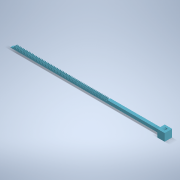
# Autodesk Inventor part: 도면
Saved by Autodesk Inventor 2021 (Build 250183000, 183)
## iProperties
Created: 2021-08-27
Part Number: 도면
Material: 티타늄
Document SubType Name: Modeling
Designer: Dongyoon
Density: 4.51 g/cm^3
Appearance: 티타늄
Author: Dongyoon
Autodesk Inventor part; units mm, degrees
ref_plane "YZ Plane" through (0, 0, 0) normal (1, 0, 0) x (0, 1, 0)
ref_plane "XZ Plane" through (0, 0, 0) normal (0, 1, 0) x (-1, 0, 0)
ref_plane "XY Plane" through (0, 0, 0) normal (0, 0, 1) x (1, 0, 0)
sketch "스케치3" plane through (0, 0, 0) normal (0, 0, 1) x (1, 0, 0)
  line L0 (0, 0) -> (0, -2)
  line L1 (0, -2) -> (-200, -2)
  line L2 (-200, -2) -> (-200, 2)
  line L3 (-200, 2) -> (0, 2)
  line L4 (0, 2) -> (0, 0)
  line L5 (-70, 2) -> (-70, -2)
  line L6 (-70, 2) -> (-71.5, 0)
  line L7 (-71.5, 0) -> (-72, 0)
  line L8 (-72, 0) -> (-72, 2)
  line L9 (-72, 2) -> (-72.5, 2)
  line L10 (-72.5, 2) -> (-73.5, 0)
  line L11 (-73.5, 0) -> (-74, 0)
  line L12 (-74, 0) -> (-74, 2)
  line L13 (-200, -2) -> (-196, 0)
  line L14 (-76, 0) -> (-76, 2)
  line L15 (-75.5, 0) -> (-76, 0)
  line L16 (-74.5, 2) -> (-75.5, 0)
  line L17 (-74, 2) -> (-74.5, 2)
  line L18 (-78, 0) -> (-78, 2)
  line L19 (-77.5, 0) -> (-78, 0)
  line L20 (-76.5, 2) -> (-77.5, 0)
  line L21 (-76, 2) -> (-76.5, 2)
  line L22 (-80, 0) -> (-80, 2)
  line L23 (-79.5, 0) -> (-80, 0)
  line L24 (-78.5, 2) -> (-79.5, 0)
  line L25 (-78, 2) -> (-78.5, 2)
  line L26 (-82, 0) -> (-82, 2)
  line L27 (-81.5, 0) -> (-82, 0)
  line L28 (-80.5, 2) -> (-81.5, 0)
  line L29 (-80, 2) -> (-80.5, 2)
  line L30 (-84, 0) -> (-84, 2)
  line L31 (-83.5, 0) -> (-84, 0)
  line L32 (-82.5, 2) -> (-83.5, 0)
  line L33 (-82, 2) -> (-82.5, 2)
  line L34 (-86, 0) -> (-86, 2)
  line L35 (-85.5, 0) -> (-86, 0)
  line L36 (-84.5, 2) -> (-85.5, 0)
  line L37 (-84, 2) -> (-84.5, 2)
  line L38 (-88, 0) -> (-88, 2)
  line L39 (-87.5, 0) -> (-88, 0)
  line L40 (-86.5, 2) -> (-87.5, 0)
  line L41 (-86, 2) -> (-86.5, 2)
  line L42 (-90, 0) -> (-90, 2)
  line L43 (-89.5, 0) -> (-90, 0)
  line L44 (-88.5, 2) -> (-89.5, 0)
  line L45 (-88, 2) -> (-88.5, 2)
  line L46 (-92, 0) -> (-92, 2)
  line L47 (-91.5, 0) -> (-92, 0)
  line L48 (-90.5, 2) -> (-91.5, 0)
  line L49 (-90, 2) -> (-90.5, 2)
  line L50 (-94, 0) -> (-94, 2)
  line L51 (-93.5, 0) -> (-94, 0)
  line L52 (-92.5, 2) -> (-93.5, 0)
  line L53 (-92, 2) -> (-92.5, 2)
  line L54 (-96, 0) -> (-96, 2)
  line L55 (-95.5, 0) -> (-96, 0)
  line L56 (-94.5, 2) -> (-95.5, 0)
  line L57 (-94, 2) -> (-94.5, 2)
  line L58 (-98, 0) -> (-98, 2)
  line L59 (-97.5, 0) -> (-98, 0)
  line L60 (-96.5, 2) -> (-97.5, 0)
  line L61 (-96, 2) -> (-96.5, 2)
  line L62 (-100, 0) -> (-100, 2)
  line L63 (-99.5, 0) -> (-100, 0)
  line L64 (-98.5, 2) -> (-99.5, 0)
  line L65 (-98, 2) -> (-98.5, 2)
  line L66 (-102, 0) -> (-102, 2)
  line L67 (-101.5, 0) -> (-102, 0)
  line L68 (-100.5, 2) -> (-101.5, 0)
  line L69 (-100, 2) -> (-100.5, 2)
  line L70 (-104, 0) -> (-104, 2)
  line L71 (-103.5, 0) -> (-104, 0)
  line L72 (-102.5, 2) -> (-103.5, 0)
  line L73 (-102, 2) -> (-102.5, 2)
  line L74 (-106, 0) -> (-106, 2)
  line L75 (-105.5, 0) -> (-106, 0)
  line L76 (-104.5, 2) -> (-105.5, 0)
  line L77 (-104, 2) -> (-104.5, 2)
  line L78 (-108, 0) -> (-108, 2)
  line L79 (-107.5, 0) -> (-108, 0)
  line L80 (-106.5, 2) -> (-107.5, 0)
  line L81 (-106, 2) -> (-106.5, 2)
  line L82 (-110, 0) -> (-110, 2)
  line L83 (-109.5, 0) -> (-110, 0)
  line L84 (-108.5, 2) -> (-109.5, 0)
  line L85 (-108, 2) -> (-108.5, 2)
  line L86 (-112, 0) -> (-112, 2)
  line L87 (-111.5, 0) -> (-112, 0)
  line L88 (-110.5, 2) -> (-111.5, 0)
  line L89 (-110, 2) -> (-110.5, 2)
  line L90 (-114, 0) -> (-114, 2)
  line L91 (-113.5, 0) -> (-114, 0)
  line L92 (-112.5, 2) -> (-113.5, 0)
  line L93 (-112, 2) -> (-112.5, 2)
  line L94 (-116, 0) -> (-116, 2)
  line L95 (-115.5, 0) -> (-116, 0)
  line L96 (-114.5, 2) -> (-115.5, 0)
  line L97 (-114, 2) -> (-114.5, 2)
  line L98 (-118, 0) -> (-118, 2)
  line L99 (-117.5, 0) -> (-118, 0)
  line L100 (-116.5, 2) -> (-117.5, 0)
  line L101 (-116, 2) -> (-116.5, 2)
  line L102 (-120, 0) -> (-120, 2)
  line L103 (-119.5, 0) -> (-120, 0)
  line L104 (-118.5, 2) -> (-119.5, 0)
  line L105 (-118, 2) -> (-118.5, 2)
  line L106 (-122, 0) -> (-122, 2)
  line L107 (-121.5, 0) -> (-122, 0)
  line L108 (-120.5, 2) -> (-121.5, 0)
  line L109 (-120, 2) -> (-120.5, 2)
  line L110 (-124, 0) -> (-124, 2)
  line L111 (-123.5, 0) -> (-124, 0)
  line L112 (-122.5, 2) -> (-123.5, 0)
  line L113 (-122, 2) -> (-122.5, 2)
  line L114 (-126, 0) -> (-126, 2)
  line L115 (-125.5, 0) -> (-126, 0)
  line L116 (-124.5, 2) -> (-125.5, 0)
  line L117 (-124, 2) -> (-124.5, 2)
  line L118 (-128, 0) -> (-128, 2)
  line L119 (-127.5, 0) -> (-128, 0)
  line L120 (-126.5, 2) -> (-127.5, 0)
  line L121 (-126, 2) -> (-126.5, 2)
  line L122 (-130, 0) -> (-130, 2)
  line L123 (-129.5, 0) -> (-130, 0)
  line L124 (-128.5, 2) -> (-129.5, 0)
  line L125 (-128, 2) -> (-128.5, 2)
  line L126 (-132, 0) -> (-132, 2)
  line L127 (-131.5, 0) -> (-132, 0)
  line L128 (-130.5, 2) -> (-131.5, 0)
  line L129 (-130, 2) -> (-130.5, 2)
  line L130 (-134, 0) -> (-134, 2)
  line L131 (-133.5, 0) -> (-134, 0)
  line L132 (-132.5, 2) -> (-133.5, 0)
  line L133 (-132, 2) -> (-132.5, 2)
  line L134 (-136, 0) -> (-136, 2)
  line L135 (-135.5, 0) -> (-136, 0)
  line L136 (-134.5, 2) -> (-135.5, 0)
  line L137 (-134, 2) -> (-134.5, 2)
  line L138 (-138, 0) -> (-138, 2)
  line L139 (-137.5, 0) -> (-138, 0)
  line L140 (-136.5, 2) -> (-137.5, 0)
  line L141 (-136, 2) -> (-136.5, 2)
  line L142 (-140, 0) -> (-140, 2)
  line L143 (-139.5, 0) -> (-140, 0)
  line L144 (-138.5, 2) -> (-139.5, 0)
  line L145 (-138, 2) -> (-138.5, 2)
  line L146 (-142, 0) -> (-142, 2)
  line L147 (-141.5, 0) -> (-142, 0)
  line L148 (-140.5, 2) -> (-141.5, 0)
  line L149 (-140, 2) -> (-140.5, 2)
  line L150 (-144, 0) -> (-144, 2)
  line L151 (-143.5, 0) -> (-144, 0)
  line L152 (-142.5, 2) -> (-143.5, 0)
  line L153 (-142, 2) -> (-142.5, 2)
  line L154 (-146, 0) -> (-146, 2)
  line L155 (-145.5, 0) -> (-146, 0)
  line L156 (-144.5, 2) -> (-145.5, 0)
  line L157 (-144, 2) -> (-144.5, 2)
  line L158 (-148, 0) -> (-148, 2)
  line L159 (-147.5, 0) -> (-148, 0)
  line L160 (-146.5, 2) -> (-147.5, 0)
  line L161 (-146, 2) -> (-146.5, 2)
  line L162 (-150, 0) -> (-150, 2)
  line L163 (-149.5, 0) -> (-150, 0)
  line L164 (-148.5, 2) -> (-149.5, 0)
  line L165 (-148, 2) -> (-148.5, 2)
  line L166 (-152, 0) -> (-152, 2)
  line L167 (-151.5, 0) -> (-152, 0)
  line L168 (-150.5, 2) -> (-151.5, 0)
  line L169 (-150, 2) -> (-150.5, 2)
  line L170 (-154, 0) -> (-154, 2)
  line L171 (-153.5, 0) -> (-154, 0)
  line L172 (-152.5, 2) -> (-153.5, 0)
  line L173 (-152, 2) -> (-152.5, 2)
  line L174 (-156, 0) -> (-156, 2)
  line L175 (-155.5, 0) -> (-156, 0)
  line L176 (-154.5, 2) -> (-155.5, 0)
  line L177 (-154, 2) -> (-154.5, 2)
  line L178 (-158, 0) -> (-158, 2)
  line L179 (-157.5, 0) -> (-158, 0)
  line L180 (-156.5, 2) -> (-157.5, 0)
  line L181 (-156, 2) -> (-156.5, 2)
  line L182 (-160, 0) -> (-160, 2)
  line L183 (-159.5, 0) -> (-160, 0)
  line L184 (-158.5, 2) -> (-159.5, 0)
  line L185 (-158, 2) -> (-158.5, 2)
  line L186 (-162, 0) -> (-162, 2)
  line L187 (-161.5, 0) -> (-162, 0)
  line L188 (-160.5, 2) -> (-161.5, 0)
  line L189 (-160, 2) -> (-160.5, 2)
  line L190 (-164, 0) -> (-164, 2)
  line L191 (-163.5, 0) -> (-164, 0)
  line L192 (-162.5, 2) -> (-163.5, 0)
  line L193 (-162, 2) -> (-162.5, 2)
  line L194 (-166, 0) -> (-166, 2)
  line L195 (-165.5, 0) -> (-166, 0)
  line L196 (-164.5, 2) -> (-165.5, 0)
  line L197 (-164, 2) -> (-164.5, 2)
  line L198 (-168, 0) -> (-168, 2)
  line L199 (-167.5, 0) -> (-168, 0)
  line L200 (-166.5, 2) -> (-167.5, 0)
  line L201 (-166, 2) -> (-166.5, 2)
  line L202 (-170, 0) -> (-170, 2)
  line L203 (-169.5, 0) -> (-170, 0)
  line L204 (-168.5, 2) -> (-169.5, 0)
  line L205 (-168, 2) -> (-168.5, 2)
  line L206 (-172, 0) -> (-172, 2)
  line L207 (-171.5, 0) -> (-172, 0)
  line L208 (-170.5, 2) -> (-171.5, 0)
  line L209 (-170, 2) -> (-170.5, 2)
  line L210 (-174, 0) -> (-174, 2)
  line L211 (-173.5, 0) -> (-174, 0)
  line L212 (-172.5, 2) -> (-173.5, 0)
  line L213 (-172, 2) -> (-172.5, 2)
  line L214 (-176, 0) -> (-176, 2)
  line L215 (-175.5, 0) -> (-176, 0)
  line L216 (-174.5, 2) -> (-175.5, 0)
  line L217 (-174, 2) -> (-174.5, 2)
  line L218 (-178, 0) -> (-178, 2)
  line L219 (-177.5, 0) -> (-178, 0)
  line L220 (-176.5, 2) -> (-177.5, 0)
  line L221 (-176, 2) -> (-176.5, 2)
  line L222 (-180, 0) -> (-180, 2)
  line L223 (-179.5, 0) -> (-180, 0)
  line L224 (-178.5, 2) -> (-179.5, 0)
  line L225 (-178, 2) -> (-178.5, 2)
  line L226 (-182, 0) -> (-182, 2)
  line L227 (-181.5, 0) -> (-182, 0)
  line L228 (-180.5, 2) -> (-181.5, 0)
  line L229 (-180, 2) -> (-180.5, 2)
  line L230 (-184, 0) -> (-184, 2)
  line L231 (-183.5, 0) -> (-184, 0)
  line L232 (-182.5, 2) -> (-183.5, 0)
  line L233 (-182, 2) -> (-182.5, 2)
  line L234 (-186, 0) -> (-186, 2)
  line L235 (-185.5, 0) -> (-186, 0)
  line L236 (-184.5, 2) -> (-185.5, 0)
  line L237 (-184, 2) -> (-184.5, 2)
  line L238 (-188, 0) -> (-188, 2)
  line L239 (-187.5, 0) -> (-188, 0)
  line L240 (-186.5, 2) -> (-187.5, 0)
  line L241 (-186, 2) -> (-186.5, 2)
  line L242 (-190, 0) -> (-190, 2)
  line L243 (-189.5, 0) -> (-190, 0)
  line L244 (-188.5, 2) -> (-189.5, 0)
  line L245 (-188, 2) -> (-188.5, 2)
  line L246 (-192, 0) -> (-192, 2)
  line L247 (-191.5, 0) -> (-192, 0)
  line L248 (-190.5, 2) -> (-191.5, 0)
  line L249 (-190, 2) -> (-190.5, 2)
  line L250 (-194, 0) -> (-194, 2)
  line L251 (-193.5, 0) -> (-194, 0)
  line L252 (-192.5, 2) -> (-193.5, 0)
  line L253 (-192, 2) -> (-192.5, 2)
  line L254 (-196, 0) -> (-196, 2)
  line L255 (-195.5, 0) -> (-196, 0)
  line L256 (-194.5, 2) -> (-195.5, 0)
  line L257 (-194, 2) -> (-194.5, 2)
  dimension "d1018" = 200
  dimension "d1019" = 4
  dimension "d1020" = 2
  dimension "d1040" = 70
  dimension "d1041" = 0.5
  dimension "d1042" = 0.5
  dimension "d1043" = 0.5
  dimension "d1044" = 2
  dimension "d1045" = 2
  dimension "d1046" = 4
  dimension "d1047" = 2
  dimension "d1050" = 2
  constraints: 514 end point, 305 horizontal alignment, 123 collinear, 122 parallel, 5 perpendicular, 4 point on line, 2 vertical, 1 horizontal, 6 other
  measures "d1018" distance of L0.end L1.end
  measures "d1019" distance of L1.end L2.end
  measures "d1020" distance of L0.start L0.end
  measures "d1040" distance between parallel lines of L4 L5
  measures "d1041" distance of L9.end L8.end
  measures "d1042" distance of L6.end L7.end
  measures "d1043" distance of L10.end L11.end
  measures "d1044" horizontal distance of L5.start L7.end
  measures "d1045" distance of L8.end L12.end
  measures "d1046" horizontal distance of L1.end L13.end
  measures "d1047" distance from line of L1 L13.end
  measures "d1050" distance of L11.end L14.start
extrude "돌출3" add sketch "스케치3" along normal mid plane 4 contours L0 L1 L5 L3 L4 | L1 L13 L255 L256 L3 L250 L251 L252 L246 L247 L248 L242 L243 L244 L238 L239 L240 L234 L235 L236 L230 L231 L232 L226 L227 L228 L222 L223 L224 L218 L219 L220 L214 L215 L216 L210 L211 L212 L206 L207 L208 L202 L203 L204 L198 L199 L200 L194 L195 L196 L190 L191 L192 L186 L187 L188 L182 L183 L184 L178 L179 L180 L174 L175 L176 L170 L171 L172 L166 L167 L168 L162 L163 L164 L158 L159 L160 L154 L155 L156 L150 L151 L152 L146 L147 L148 L142 L143 L144 L138 L139 L140 L134 L135 L136 L130 L131 L132 L126 L127 L128 L122 L123 L124 L118 L119 L120 L114 L115 L116 L110 L111 L112 L106 L107 L108 L102 L103 L104 L98 L99 L100 L94 L95 L96 L90 L91 L92 L86 L87 L88 L82 L83 L84 L78 L79 L80 L74 L75 L76 L70 L71 L72 L66 L67 L68 L62 L63 L64 L58 L59 L60 L54 L55 L56 L50 L51 L52 L46 L47 L48 L42 L43 L44 L38 L39 L40 L34 L35 L36 L30 L31 L32 L26 L27 L28 L22 L23 L24 L18 L19 L20 L14 L15 L16 L12 L11 L10 L8 L7 L6 L5
sketch "스케치4" plane through (0, 0, 0) normal (0, 0, 1) x (1, 0, 0)
  line L0 (0, 0) -> (0, 5)
  line L1 (0, 5) -> (10, 5)
  line L2 (10, 5) -> (10, -5)
  line L3 (10, -5) -> (0, -5)
  line L4 (0, -5) -> (0, 0)
  line L5 (0, -2) -> (0, 2) projected
  dimension "d1023" = 10
  dimension "d1024" = 10
  dimension "d1025" = 5
  constraints: 10 end point, 3 perpendicular, 1 collinear, 1 point on line, 1 vertical
  measures "d1023" distance of L1.end L2.end
  measures "d1024" distance of L2.end L3.end
  measures "d1025" distance of L3.end L0.start
extrude "돌출4" add sketch "스케치4" along normal mid plane 10
sketch "스케치6" plane through (0, 0, 0) normal (0, 0, 1) x (1, 0, 0)
  line L0 (0, 5) -> (10, 5) projected
  line L1 (10, -5) -> (0, -5) projected
  line L2 (3, 5) -> (7, 5)
  line L3 (7, 5) -> (7, -5)
  line L4 (7, -5) -> (3, -5)
  line L5 (3, -5) -> (3, 5)
  line L6 (0, -5) -> (0, 5) projected
  line L7 (3, 5) -> (5, 4)
  line L8 (5, 4) -> (5, 3.5)
  line L9 (5, 3.5) -> (3, 3.5)
  line L10 (3, 3.5) -> (3, 3)
  line L11 (3, 3) -> (5, 2)
  line L12 (5, 2) -> (5, 1.5)
  line L13 (5, 1.5) -> (3, 1.5)
  line L14 (3, 1.5) -> (3, 1)
  line L15 (3, 1) -> (5, 0)
  line L16 (5, 0) -> (5, -0.5)
  line L17 (5, -0.5) -> (3, -0.5)
  line L18 (3, -0.5) -> (3, -1)
  line L19 (3, -1) -> (5, -2)
  line L20 (5, -2) -> (5, -2.5)
  line L21 (5, -2.5) -> (3, -2.5)
  line L22 (3, -2.5) -> (3, -3)
  line L23 (3, -3) -> (5, -4)
  line L24 (5, -4) -> (5, -4.5)
  line L25 (5, -4.5) -> (3, -4.5)
  point P0 (0, 0)
  dimension "d1055" = 3
  dimension "d1056" = 4
  dimension "d1057" = 0.5
  dimension "d1058" = 0.5
  dimension "d1059" = 0.5
  dimension "d1060" = 2
  dimension "d1061" = 2
  dimension "d1062" = 2
  dimension "d1063" = 0.5
  dimension "d1064" = 0.5
  dimension "d1065" = 0.5
  dimension "d1066" = 0.5
  dimension "d1067" = 0.5
  dimension "d1068" = 0.5
  constraints: 46 end point, 7 point on line, 3 perpendicular, 2 parallel, 1 horizontal, 1 vertical
  measures "d1055" distance between parallel lines of L6 L5
  measures "d1056" distance between parallel lines of L5 L3
  measures "d1057" distance of L7.end L8.end
  measures "d1058" distance of L9.end L10.end
  measures "d1059" distance of L11.end L12.end
  measures "d1060" distance of L10.end L2.start
  measures "d1061" distance of L11.end L7.end
  measures "d1062" distance between parallel lines of L3 L8
  measures "d1063" distance of L14.start L14.end
  measures "d1064" distance of L15.end L16.end
  measures "d1065" distance of L18.start L18.end
  measures "d1066" distance of L19.end L20.end
  measures "d1067" distance of L22.start L22.end
  measures "d1068" distance of L23.end L24.end
extrude "돌출5" cut sketch "스케치6" against normal mid plane 4 contours L0 L3 L1 L5 L25 L24 L23 L21 L20 L19 L17 L16 L15 L13 L12 L11 L9 L8 L7
